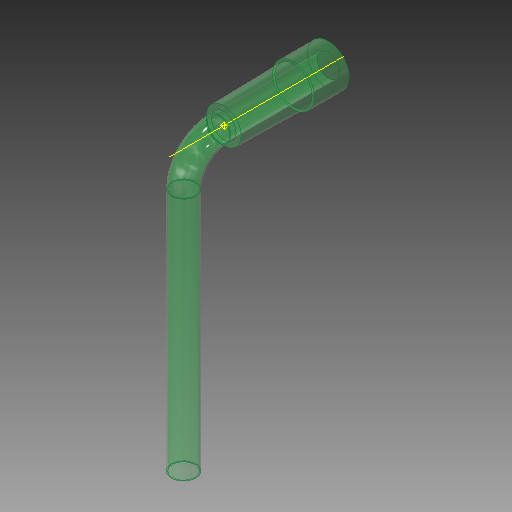
# Autodesk Inventor part: Tubo de Entrada do Ar
Saved by Autodesk Inventor 2019 (Build 230136000, 136)
## iProperties
Created: 2020-04-02
Part Number: Tubo de Entrada do Ar
Material: Genérico
Document SubType Name: Modeling
Designer: Paulo Rodrigues
Density: 1 g/cm^3
Appearance: Transparente - Verde 1
Author: Paulo Rodrigues
Autodesk Inventor part; units mm, degrees
ref_plane "YZ Plane" through (0, 0, 0) normal (1, 0, 0) x (0, 1, 0)
ref_plane "XZ Plane" through (0, 0, 0) normal (0, 1, 0) x (-1, 0, 0)
ref_plane "XY Plane" through (0, 0, 0) normal (0, 0, 1) x (1, 0, 0)
sketch "Esboço1" plane through (0, 0, 0) normal (0, 0, 1) x (1, 0, 0)
  circle A0 centre (0, 0) radius 3.25 projected
  circle A1 centre (0, 0) radius 6
  point P0 (0, 0)
  dimension "d0" = 12
  constraints: 1 centre point
  measures "d0" diameter of A1
extrude "Extrusão1" add sketch "Esboço1" along normal mid plane 10
sketch "Esboço2" plane through (0, 0, 5) normal (0, 0, 1) x (1, 0, 0)
  circle A0 centre (0, 0) radius 6 projected
  circle A1 centre (0, 0) radius 5
  circle A2 centre (0, 0) radius 3.25 projected
  point P0 (0, 0)
  dimension "d3" = 1
  constraints: 1 centre point
  measures "d3" radial gap between concentric circles of A0 A1
extrude "Extrusão2" add sketch "Esboço2" along normal blind 20 contours A1
draft "Face para inclinação de faces1" angle 1 pull direction (0, 0, 1) faces at (4.9353, -0.8021, 18.3333) fixed edges at (-5, 0, 25)
sketch "Esboço3" plane through (0, 0, 25) normal (0, 0, 1) x (1, 0, 0)
  circle A0 centre (0, 0) radius 3.25 projected
  circle A1 centre (0, 0) radius 3.55
  point P0 (0, 0)
  dimension "d7" = 0.3
  constraints: 1 centre point
  measures "d7" radial gap between concentric circles of A1 A0
sketch3d "Esboço 3D1"
  line L0 (0, 0, 25) -> (0, 0, 26.4983)
  arc A0 (0, 0, 26.4983) -> (0, -10, 36.4983) centre (0, -10, 26.4983) ccw
  line L1 (0, -10, 36.4983) -> (0, -80, 36.4983)
  dimension "d8" = 80
  dimension "d9" = 10
sweep "Varredura1" add profiles "Esboço3" path "Esboço 3D1"
